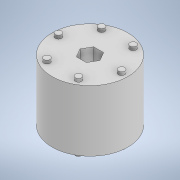
# Autodesk Inventor part: new mech inside
Saved by Autodesk Inventor 2020.2 (Build 242310000, 310)
## iProperties
Created: 2020-04-13
Part Number: new mech inside
Material: Generic
Document SubType Name: Modeling
Designer: deli
Density: 1 g/cm^3
Appearance: Default
Author: deli
Autodesk Inventor part; units mm, degrees
ref_plane "YZ Plane" through (0, 0, 0) normal (1, 0, 0) x (0, 1, 0)
ref_plane "XZ Plane" through (0, 0, 0) normal (0, 1, 0) x (-1, 0, 0)
ref_plane "XY Plane" through (0, 0, 0) normal (0, 0, 1) x (1, 0, 0)
sketch "Sketch1" plane through (0, 0, 0) normal (0, 1, 0) x (-1, 0, 0)
  circle A0 centre (0, 0) radius 28.5
  circle A1 centre (0, 0) radius 9
  circle A2 centre (11.875, 20.5681) radius 1.5875
  circle A3 centre (-11.875, 20.5681) radius 1.5875
  circle A4 centre (23.75, 0) radius 1.5875
  circle A5 centre (11.875, -20.5681) radius 1.5875
  circle A6 centre (-11.875, -20.5681) radius 1.5875
  circle A7 centre (-23.75, 0) radius 1.5875
  dimension "d5" = 3.175
  dimension "d6" = 20.5681
  dimension "d7" = 3.175
  dimension "d8" = 3.175
  dimension "d9" = 3.175
  dimension "d10" = 3.175
  dimension "d11" = 3.175
  constraints: 8 centre point, 2 other
  measures "d5" diameter of A5
  measures "d6" vertical distance of A0.centre A5.centre
  measures "d7" diameter of A6
  measures "d8" diameter of A7
  measures "d9" diameter of A3
  measures "d10" diameter of A2
  measures "d11" diameter of A4
extrude "Extrusion1" add sketch "Sketch1" along normal blind 46
sketch "Sketch2" plane through (0, 46, 0) normal (0, 1, 0) x (1, 0, 0)
  line L0 (7.5157, 0) -> (3.7578, -6.5088)
  line L1 (3.7578, -6.5088) -> (-3.7578, -6.5088)
  line L2 (-3.7578, -6.5088) -> (-7.5157, 0)
  line L3 (-7.5157, 0) -> (-3.7578, 6.5088)
  line L4 (-3.7578, 6.5088) -> (3.7578, 6.5088)
  line L5 (3.7578, 6.5088) -> (7.5157, 0)
  circle A0 centre (0, 0) radius 28.5 projected
  circle A1 centre (-11.875, -20.5681) radius 1.5875 projected
  circle A2 centre (11.875, -20.5681) radius 1.5875 projected
  circle A3 centre (-23.75, 0) radius 1.5875 projected
  circle A4 centre (-11.875, 20.5681) radius 1.5875 projected
  circle A5 centre (23.75, 0) radius 1.5875 projected
  circle A6 centre (11.875, 20.5681) radius 1.5875 projected
  dimension "d4" = 13.0175
  constraints: 12 end point, 7 centre point
  measures "d4" distance between parallel lines of L1 L4
extrude "Extrusion2" add sketch "Sketch2" against normal blind 46
sketch "Sketch3" plane through (0, 46, 0) normal (0, 1, 0) x (1, 0, 0)
  circle A0 centre (-11.875, 20.5681) radius 1.5875 projected
  circle A1 centre (-11.875, 20.5681) radius 2.3812
  circle A2 centre (11.875, 20.5681) radius 1.5875 projected
  circle A3 centre (11.875, 20.5681) radius 2.3812
  circle A4 centre (23.75, 0) radius 1.5875 projected
  circle A5 centre (23.75, 0) radius 2.3813
  circle A6 centre (11.875, -20.5681) radius 1.5875 projected
  circle A7 centre (11.875, -20.5681) radius 2.3813
  circle A8 centre (-11.875, -20.5681) radius 1.5875 projected
  circle A9 centre (-11.875, -20.5681) radius 2.3812
  circle A10 centre (-23.75, 0) radius 1.5875 projected
  circle A11 centre (-23.75, 0) radius 2.3812
  point P0 (0, 0)
  dimension "d12" = 4.7625
  dimension "d13" = 4.7625
  dimension "d14" = 4.7625
  dimension "d15" = 4.7625
  dimension "d16" = 4.7625
  dimension "d17" = 4.7625
  constraints: 6 centre point, 6 coincident
  measures "d12" diameter of A1
  measures "d13" diameter of A3
  measures "d14" diameter of A5
  measures "d15" diameter of A7
  measures "d16" diameter of A9
  measures "d17" diameter of A11
extrude "Extrusion3" add sketch "Sketch3" along normal blind 2.3813 and the other way blind 48.3807 contours A0 | A1 | A2 | A3 | A4 | A5 | A6 | A7 | A8 | A9 | A10 | A11
equation "\"d7\" = d5"
equation "\"d8\" = d5"
equation "\"d9\" = d5"
equation "\"d10\" = d5"
equation "\"d11\" = d5"
body "Solid1"
